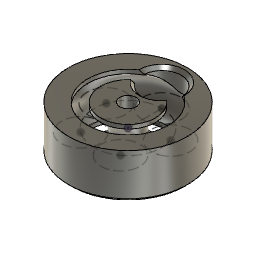
TestBearings v10 (Autodesk Fusion 360 design; units mm, degrees)
Autodesk Fusion 360 part; units mm, degrees
note: some values were not read from the file. Set by a fixed rule: which sketch regions a step uses.
sketch "Sketch4" plane through (0, 0, 0) normal (0, 0, 1) x (1, 0, 0) in component "Bearing"
  circle A0 centre (0, 0) radius 1.274
  circle A1 centre (0, 0) radius 4.274
  circle A2 centre (0, 0) radius 6.274
  circle A3 centre (0, 0) radius 9.274
  dimension "d27" = 2.5481
  dimension "d28" = 8.5481
  dimension "d29" = 12.5481
  dimension "d30" = 18.5481
  constraint concentric A0 A1
  constraint concentric A0 A2
  constraint concentric A2 A3
  constraint coincident A0.centre A1.centre
  measures "d27" diameter of A0
  measures "d28" diameter of A1
  measures "d29" diameter of A2
  measures "d30" diameter of A3
extrude "Extrude3" add sketch "Sketch4" along normal blind 7 makes body 1 at (4.2528, -0.4256, 4.6667) makes body 2 at (9.2625, -0.4623, 2.3333) in component "Bearing"
sketch "Sketch5" plane through (0, 0, 0) normal (0, 1, 0) x (1, 0, 0) in component "Bearing"
  line L0 (1.274, -7) -> (-1.274, -7) construction
  line L1 (1.274, 0) -> (-1.274, 0) construction
  line L2 (0, -7) -> (0, 0) construction
  line L3 (-5.274, -7) -> (-5.274, 0) construction
  circle A0 centre (-5.274, -3.5) radius 3.05
  dimension "d33" = 5.274
  dimension "d34" = 6.1
  constraint midpoint L0 L2.start
  constraint midpoint L1 L2.end
  constraint coincident L0 L3.start
  constraint coincident L1 L3.end
  constraint perpendicular L1 L3
  constraint midpoint L3 A0.centre
  measures "d33" distance of L2 L3
  measures "d34" diameter of A0
revolve "Revolve2" cut sketch "Sketch5" angle 360 about axis through (0, 0, 7) along (0, 0, -1) bodies 1 2 in component "Bearing"
sketch "Sketch6" plane through (0, 0, 7) normal (0, 0, 1) x (-1, 0, 0) in component "Bearing"
  circle A0 centre (0, 0) radius 6.274
  circle A1 centre (0, 0) radius 9.274
  line L0 (0, 0) -> (0, -9.274) construction
  circle A2 centre (0, -5.274) radius 3
  dimension "d36" = 9.274
  dimension "d37" = 6
  dimension "d38" = 5.274
  constraint coincident A0.centre A1.centre
  constraint vertical L0
  constraint coincident L0 A2.centre
  measures "d36" distance of A0.centre L0.end
  measures "d37" diameter of A2
  measures "d38" distance of A0.centre A2.centre
extrude "Extrude4" cut sketch "Sketch6" against normal blind 3.5 contours A0 A2 | A0 A2 picked at (-0.0403, -4.931) picked at (0, -6.9302) bodies 1 2 in component "Bearing"
chamfer "Chamfer2" distance 0.5 angle 45 2 edges at (0, 8.274, 7) (0, 2.274, 7) on bodies 1 2 in component "Bearing"
chamfer "Chamfer3" distance 0.5 angle 45 2 edges at (-8.6464, -3.3536, 0) (-1.1878, 0.4607, 0) on bodies 1 2 in component "Bearing"
ref_plane "WorkPlane1" through (0, 0, 3.5) normal (0, 0, 1) x (1, 0, 0) in component "Bearing"
sketch "Sketch7" plane through (0, 0, 3.5) normal (0, 0, 1) x (1, 0, 0) in component "Bearing"
  circle A0 centre (0, 0) radius 5.274 construction
  line L0 (0, 0) -> (0, 5.274) construction
  circle A1 centre (0, 5.274) radius 3 construction
  circle A2 centre (-5.0159, 1.6298) radius 3 construction
  circle A3 centre (-3.1, -4.2668) radius 3 construction
  circle A4 centre (3.1, -4.2668) radius 3 construction
  circle A5 centre (5.0159, 1.6298) radius 3 construction
  dimension "d45" = 10.5481
  dimension "d46" = 6
  dimension "d48" = 360
  constraint coincident A0.centre L0.start
  constraint coincident A0 L0.end
  constraint vertical L0
  constraint coincident L0.end A1.centre
  measures "d45" diameter of A0
  measures "d46" diameter of A1
component "Bearing" placed x (1, 0, 0) y (0, 1, 0) z (0, 0, 1) at (0, 0, 0)
equation "d = 6 mm" comment "ball dia"
equation "gap = 0.2 mm" comment "gap between balls"
equation "Nball = 5" comment "number of balls"
equation "D = ( d + 5 * gap / Nball ) / sin(( 180 / Nball ) * 1 deg)" comment "diameter of the ball to stay"
equation "innerinner = D - d - 2 mm"
equation "innerouter = D - 2 mm"
equation "outerinner = D + 2 mm"
equation "outerouter = D + d + 2 mm"
equation "d27 = innerinner"
equation "d28 = innerouter"
equation "d29 = outerinner"
equation "d30 = outerouter"
equation "d31 = height"
equation "d33 = D / 2"
equation "d34 = d + gap / 2"
equation "d36 = outerouter / 2"
equation "d37 = d"
equation "d38 = D / 2"
equation "height = 7 mm"
equation "d40 = -height / 2"
equation "d44 = height / 2"
equation "d45 = D"
equation "d46 = d"
equation "d47 = Nball"
